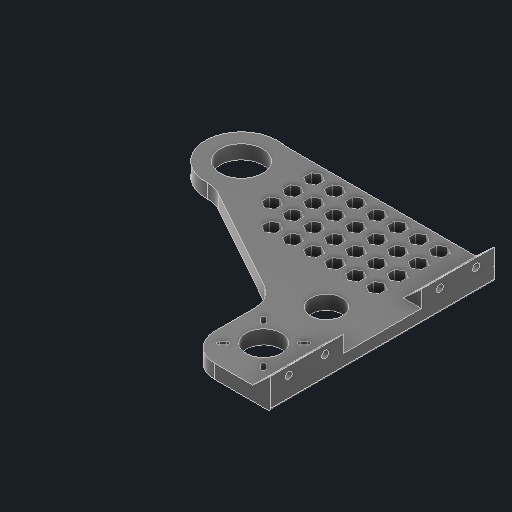
# Autodesk Inventor part: Holder
Saved by Autodesk Inventor 2023 (Build 270158000, 158)
## iProperties
Created: 2023-11-13
Part Number: Holder
Material: Acetal Resin, Black
Document SubType Name: Modeling
Designer: danie
Density: 1.425 g/cm^3
Appearance: Smooth - Black
Author: danie
Autodesk Inventor part; units mm, degrees
ref_plane "YZ Plane" through (0, 0, 0) normal (1, 0, 0) x (0, 1, 0)
ref_plane "XZ Plane" through (0, 0, 0) normal (0, 1, 0) x (-1, 0, 0)
ref_plane "XY Plane" through (0, 0, 0) normal (0, 0, 1) x (1, 0, 0)
sketch "Sketch1" plane through (0, 0, 0) normal (0, 1, 0) x (-1, 0, 0)
  circle A0 centre (35, -30) radius 12.6754
  line L0 (47.071, -15.7062) -> (49.606, -13.1712)
  arc A1 (47.071, -15.7062) -> (49.301, -17.9217) centre (48.1824, -16.8176) ccw
  line L1 (51.8288, -15.394) -> (49.301, -17.9217)
  arc A2 (51.8288, -15.394) -> (49.606, -13.1712) centre (50.7174, -14.2826) ccw
  arc A3 (20.394, -13.1712) -> (18.2539, -15.471) centre (19.2826, -14.2826) ccw
  line L2 (20.394, -13.1712) -> (22.929, -15.7062)
  line L3 (20.6292, -17.8463) -> (18.2539, -15.471)
  arc A4 (20.6292, -17.8463) -> (22.929, -15.7062) centre (21.8176, -16.8176) ccw
  arc A5 (22.929, -44.2938) -> (20.7062, -42.071) centre (21.8176, -43.1824) ccw
  line L4 (22.929, -44.2938) -> (20.394, -46.8288)
  line L5 (18.1712, -44.606) -> (20.7062, -42.071)
  arc A6 (18.1712, -44.606) -> (20.394, -46.8288) centre (19.2826, -45.7174) ccw
  arc A7 (49.606, -46.8288) -> (51.8288, -44.606) centre (50.7174, -45.7174) ccw
  line L6 (49.2938, -42.071) -> (51.8288, -44.606)
  line L7 (49.606, -46.8288) -> (47.071, -44.2938)
  arc A8 (49.2938, -42.071) -> (47.071, -44.2938) centre (48.1824, -43.1824) ccw
  line L8 (0, 0) -> (60, 0)
  line L9 (60, 0) -> (60, -120)
  line L10 (60, -120) -> (0, -120)
  line L11 (0, -120) -> (0, 0)
  line L12 (60, -60) -> (0, -60)
  line L13 (60, -60) -> (150, -110)
  line L14 (150, -110) -> (150, -160)
  line L15 (150, -160) -> (0, -160)
  line L16 (0, -160) -> (0, -120)
  arc A9 (150, -160) -> (150, -110) centre (155.9349, -135) ccw
  circle A10 centre (155.9349, -135) radius 15.25
  line L17 (35, -30) -> (35, -120)
  circle A11 centre (35, -75) radius 11.25
  point P0 (35, -30)
  point P1 (150, -135)
  point P2 (0, -140)
  point P3 (30, -60)
  dimension "d0" = 60
  dimension "d1" = 120
  dimension "d2" = 13.1824
  dimension "d3" = 15.7174
  dimension "d4" = 13.1824
  dimension "d5" = 15.7174
  dimension "d6" = 13.1824
  dimension "d7" = 15.7174
  dimension "d8" = 13.1824
  dimension "d9" = 15.7174
  dimension "d10" = 13.1824
  dimension "d11" = 15.7174
  dimension "d12" = 13.1824
  dimension "d13" = 15.7174
  dimension "d14" = 13.1824
  dimension "d15" = 15.7174
  dimension "d16" = 13.1824
  dimension "d17" = 15.7174
  dimension "d18" = 30
  dimension "d19" = 25
  dimension "d20" = 50
  dimension "d21" = 150
  dimension "d22" = 30.5
  dimension "d90" = 50
  dimension "d91" = 15
  dimension "d92" = 22.5
  dimension "d101" = 120.9349
  dimension "d102" = 35
  dimension "d103" = 135.001
  dimension "d104" = 60
  dimension "d105" = 155.9349
  constraints: 36 end point, 18 point on circle, 12 centre point, 7 midpoint, 4 perpendicular, 2 parallel, 1 coincident, 1 horizontal, 1 point on line, 1 vertical
  measures "d0" distance between parallel lines of L11 L9
  measures "d1" distance between parallel lines of L10 L8
  measures "d2" horizontal distance of A1.centre point (35, -30)
  measures "d3" horizontal distance of A2.centre point (35, -30)
  measures "d4" horizontal distance of A8.centre point (35, -30)
  measures "d5" horizontal distance of A7.centre point (35, -30)
  measures "d6" horizontal distance of A5.centre point (35, -30)
  measures "d7" horizontal distance of A6.centre point (35, -30)
  measures "d8" horizontal distance of A4.centre point (35, -30)
  measures "d9" horizontal distance of A3.centre point (35, -30)
  measures "d10" horizontal distance of A1.centre point (35, -30)
  measures "d11" horizontal distance of A2.centre point (35, -30)
  measures "d12" horizontal distance of A8.centre L17.start
  measures "d13" horizontal distance of point (35, -30) A7.centre
  measures "d14" horizontal distance of A5.centre point (35, -30)
  measures "d15" horizontal distance of A6.centre point (35, -30)
  measures "d16" horizontal distance of A4.centre point (35, -30)
  measures "d17" horizontal distance of A3.centre point (35, -30)
  measures "d18" distance from line of L12 point (35, -30)
  measures "d19" distance from line of point (35, -30) L9
  measures "d20" distance of L13.end L14.end
  measures "d21" distance from line of L16 point (150, -135)
  measures "d22" diameter of A10
  measures "d90" vertical distance of L12.start L13.end
  measures "d91" vertical distance of point (30, -60) A11.centre
  measures "d92" diameter of A11
  measures "d101" horizontal distance of point (35, -75) A9.centre
  measures "d102" distance from line of L11 point (35, -75)
  measures "d103" distance of A11.centre A9.centre
  measures "d104" vertical distance of A11.centre A10.centre
  measures "d105" distance from line of L16 A10.centre
extrude "Extrusion1" add sketch "Sketch1" along normal blind 10 contours L12 L11 L8 L9 | L12 L9 L10 L17 A11 | L17 A11 L10 L11 L12 | L13 L14 A10 L15 L16 L10 L9 | A9 L14 A10
fillet "Fillet1" radius 20 4 edges at (-60, 5, -60) (-60, 5, 0) (-150, 5, -110) (-150, 5, -160)
sketch "Sketch2" plane through (0, 0, 0) normal (0, 0, 1) x (1, 0, 0)
  line L0 (-40, 0) -> (-40, 10) projected
  line L1 (-40, 0) -> (0, 0) projected
  line L2 (0, 0) -> (0, 10) projected
  line L3 (-40, 10) -> (0, 10) projected
  line L4 (0, 10) -> (0, 22)
  line L5 (-20.6292, 0) -> (-18.2539, 0) projected
  line L6 (-18.2539, 0) -> (-18.2539, 10) projected
  line L7 (-20.6292, 10) -> (-18.2539, 10) projected
  line L8 (-20.6292, 0) -> (-20.6292, 10) projected
  line L9 (0, 22) -> (-13, 10)
  line L10 (0, 10) -> (-147.9967, 10) projected
  dimension "d26" = 12
  dimension "d28" = 13
  constraints: 4 end point, 1 point on line, 1 vertical
  measures "d26" distance of L2.end L4.end
  measures "d28" horizontal distance of L4.end L9.end
extrude "Extrusion2" add sketch "Sketch2" against normal blind 160.25 contours L9 L4 L3
sketch "Sketch3" plane through (0, 10, 0) normal (0, 1, 0) x (1, 0, 0)
  line L0 (0, 0) -> (-13, 0) projected
  line L1 (0, 0) -> (0, 160.25) projected
  line L2 (-13, 160.25) -> (0, 160.25) projected
  line L3 (-13, 0) -> (-13, 160) projected
  line L4 (-13, 80) -> (0, 80.125)
  line L5 (-13, 80) -> (-13, 52)
  line L6 (-13, 52) -> (0, 52)
  line L7 (0, 80.125) -> (0, 52)
  line L8 (0, 0) -> (0, 160.25) projected
  line L9 (-13, 80) -> (-13, 108)
  line L10 (-13, 108) -> (0, 108)
  line L11 (0, 108) -> (0, 80.125)
  line L12 (-13, 160) -> (-13, 160.25) projected
  dimension "d31" = 28
  dimension "d32" = 28
  constraints: 14 end point, 4 point on line, 2 collinear, 2 midpoint, 2 perpendicular
  measures "d31" distance of L4.start L5.end
  measures "d32" distance of L4.start L9.end
extrude "Extrusion3" cut sketch "Sketch3" along normal blind 170 contours L6 L3 L4 L1 | L4 L3 L10 L1
sketch "Sketch4" plane through (0, 0, 0) normal (1, 0, 0) x (0, 0, -1)
  line L0 (52, 22) -> (52, 10) projected
  line L1 (52, 16) -> (0, 16)
  line L2 (0, 0) -> (0, 22) projected
  line L3 (108, 10) -> (108, 22) projected
  line L4 (160.25, 10) -> (160.25, 22) projected
  line L5 (0, 22) -> (52, 22) projected
  line L6 (26, 22) -> (26, 16)
  line L7 (108, 22) -> (160.25, 22) projected
  line L8 (26, 16) -> (0, 16)
  line L9 (26, 16) -> (52, 16)
  circle A0 centre (13, 16) radius 2.5
  circle A1 centre (39, 16) radius 2.5
  circle A2 centre (121.1563, 16) radius 2.5
  circle A3 centre (147.2188, 16) radius 2.5
  line L10 (108, 22) -> (108, 10) projected
  line L11 (108, 16) -> (160.25, 16)
  line L12 (134.125, 22) -> (134.125, 16)
  point P0 (170, 12)
  dimension "d35" = 5
  dimension "d36" = 5
  dimension "d37" = 5
  dimension "d84" = 6
  dimension "d85" = 6
  constraints: 12 end point, 9 midpoint, 4 centre point, 3 point on line, 2 collinear, 1 horizontal, 2 other
  measures "d35" diameter of A0
  measures "d36" diameter of A1
  measures "d37" diameter of A2
  measures "d84" distance of point (26, 22) L6.end
  measures "d85" distance between parallel lines of L5 L1
extrude "Extrusion4" cut sketch "Sketch4" against normal blind 170 contours A1 L1 | L1 A1 | A0 L1 | L1 A0 | L11 A2 | A2 L11 | L11 A3 | A3 L11
chamfer "Chamfer1" distance 2 angle 45 4 edges at (-6.5, 16, -10.5) (-6.5, 16, -36.5) (-6.5, 16, -118.6563) (-6.5, 16, -144.7188)
sketch "Sketch5" plane through (0, 10, 0) normal (0, 1, 0) x (1, 0, 0)
  arc A0 (-151.4711, 160.3041) -> (-154.8498, 109.3281) centre (-155.9349, 135) ccw projected
  line L0 (0, 160) -> (-147.9967, 160) projected
  line L1 (-147.9967, 160) -> (0, 160)
  line L2 (-73.9983, 160) -> (-73.9983, 67.7769)
  line L3 (-144.2924, 106.8291) -> (-70.2871, 65.7151) projected
  circle A1 centre (-155.9349, 135) radius 15.25 projected
  line L4 (-140.6849, 135) -> (-73.9983, 135)
  line L5 (-73.9983, 135) -> (0, 135)
  line L6 (0, 0) -> (0, 160) projected
  line L7 (-73.9983, 140.4872) -> (-69.2463, 137.7436)
  line L8 (-69.2463, 137.7436) -> (-69.2463, 132.2564)
  line L9 (-69.2463, 132.2564) -> (-73.9983, 129.5128)
  line L10 (-73.9983, 129.5128) -> (-78.7504, 132.2564)
  line L11 (-78.7504, 132.2564) -> (-78.7504, 137.7436)
  line L12 (-78.7504, 137.7436) -> (-73.9983, 140.4872)
  line L13 (-73.9983, 125.4872) -> (-69.2463, 122.7436)
  line L14 (-69.2463, 122.7436) -> (-69.2463, 117.2564)
  line L15 (-69.2463, 117.2564) -> (-73.9983, 114.5128)
  line L16 (-73.9983, 114.5128) -> (-78.7504, 117.2564)
  line L17 (-78.7504, 122.7436) -> (-73.9983, 125.4872)
  line L18 (-78.7504, 117.2564) -> (-78.7504, 122.7436)
  line L19 (-73.9983, 110.4872) -> (-69.2463, 107.7436)
  line L20 (-69.2463, 107.7436) -> (-69.2463, 102.2564)
  line L21 (-69.2463, 102.2564) -> (-73.9983, 99.5128)
  line L22 (-73.9983, 99.5128) -> (-78.7504, 102.2564)
  line L23 (-78.7504, 107.7436) -> (-73.9983, 110.4872)
  line L24 (-78.7504, 102.2564) -> (-78.7504, 107.7436)
  line L25 (-88.9983, 140.4872) -> (-84.2463, 137.7436)
  line L26 (-84.2463, 137.7436) -> (-84.2463, 132.2564)
  line L27 (-84.2463, 132.2564) -> (-88.9983, 129.5128)
  line L28 (-88.9983, 129.5128) -> (-93.7504, 132.2564)
  line L29 (-93.7504, 137.7436) -> (-88.9983, 140.4872)
  line L30 (-93.7504, 132.2564) -> (-93.7504, 137.7436)
  line L31 (-88.9983, 125.4872) -> (-84.2463, 122.7436)
  line L32 (-84.2463, 122.7436) -> (-84.2463, 117.2564)
  line L33 (-84.2463, 117.2564) -> (-88.9983, 114.5128)
  line L34 (-88.9983, 114.5128) -> (-93.7504, 117.2564)
  line L35 (-93.7504, 122.7436) -> (-88.9983, 125.4872)
  line L36 (-93.7504, 117.2564) -> (-93.7504, 122.7436)
  line L37 (-88.9983, 110.4872) -> (-84.2463, 107.7436)
  line L38 (-84.2463, 107.7436) -> (-84.2463, 102.2564)
  line L39 (-84.2463, 102.2564) -> (-88.9983, 99.5128)
  line L40 (-88.9983, 99.5128) -> (-93.7504, 102.2564)
  line L41 (-93.7504, 107.7436) -> (-88.9983, 110.4872)
  line L42 (-93.7504, 102.2564) -> (-93.7504, 107.7436)
  line L43 (-103.9983, 140.4872) -> (-99.2463, 137.7436)
  line L44 (-99.2463, 137.7436) -> (-99.2463, 132.2564)
  line L45 (-99.2463, 132.2564) -> (-103.9983, 129.5128)
  line L46 (-103.9983, 129.5128) -> (-108.7504, 132.2564)
  line L47 (-108.7504, 137.7436) -> (-103.9983, 140.4872)
  line L48 (-108.7504, 132.2564) -> (-108.7504, 137.7436)
  line L49 (-103.9983, 125.4872) -> (-99.2463, 122.7436)
  line L50 (-99.2463, 122.7436) -> (-99.2463, 117.2564)
  line L51 (-99.2463, 117.2564) -> (-103.9983, 114.5128)
  line L52 (-103.9983, 114.5128) -> (-108.7504, 117.2564)
  line L53 (-108.7504, 122.7436) -> (-103.9983, 125.4872)
  line L54 (-108.7504, 117.2564) -> (-108.7504, 122.7436)
  line L55 (-103.9983, 110.4872) -> (-99.2463, 107.7436)
  line L56 (-99.2463, 107.7436) -> (-99.2463, 102.2564)
  line L57 (-99.2463, 102.2564) -> (-103.9983, 99.5128)
  line L58 (-103.9983, 99.5128) -> (-108.7504, 102.2564)
  line L59 (-108.7504, 107.7436) -> (-103.9983, 110.4872)
  line L60 (-108.7504, 102.2564) -> (-108.7504, 107.7436)
  line L61 (-78.7504, 152.7436) -> (-73.9983, 155.4872)
  line L62 (-78.7504, 147.2564) -> (-78.7504, 152.7436)
  line L63 (-73.9983, 144.5128) -> (-78.7504, 147.2564)
  line L64 (-69.2463, 147.2564) -> (-73.9983, 144.5128)
  line L65 (-69.2463, 152.7436) -> (-69.2463, 147.2564)
  line L66 (-73.9983, 155.4872) -> (-69.2463, 152.7436)
  line L67 (-63.7504, 137.7436) -> (-58.9983, 140.4872)
  line L68 (-63.7504, 132.2564) -> (-63.7504, 137.7436)
  line L69 (-58.9983, 129.5128) -> (-63.7504, 132.2564)
  line L70 (-54.2463, 132.2564) -> (-58.9983, 129.5128)
  line L71 (-54.2463, 137.7436) -> (-54.2463, 132.2564)
  line L72 (-58.9983, 140.4872) -> (-54.2463, 137.7436)
  line L73 (-63.7504, 152.7436) -> (-58.9983, 155.4872)
  line L74 (-63.7504, 147.2564) -> (-63.7504, 152.7436)
  line L75 (-58.9983, 144.5128) -> (-63.7504, 147.2564)
  line L76 (-54.2463, 147.2564) -> (-58.9983, 144.5128)
  line L77 (-54.2463, 152.7436) -> (-54.2463, 147.2564)
  line L78 (-58.9983, 155.4872) -> (-54.2463, 152.7436)
  line L79 (-48.7504, 137.7436) -> (-43.9983, 140.4872)
  line L80 (-48.7504, 132.2564) -> (-48.7504, 137.7436)
  line L81 (-43.9983, 129.5128) -> (-48.7504, 132.2564)
  line L82 (-39.2463, 132.2564) -> (-43.9983, 129.5128)
  line L83 (-39.2463, 137.7436) -> (-39.2463, 132.2564)
  line L84 (-43.9983, 140.4872) -> (-39.2463, 137.7436)
  line L85 (-48.7504, 152.7436) -> (-43.9983, 155.4872)
  line L86 (-48.7504, 147.2564) -> (-48.7504, 152.7436)
  line L87 (-43.9983, 144.5128) -> (-48.7504, 147.2564)
  line L88 (-39.2463, 147.2564) -> (-43.9983, 144.5128)
  line L89 (-39.2463, 152.7436) -> (-39.2463, 147.2564)
  line L90 (-43.9983, 155.4872) -> (-39.2463, 152.7436)
  line L91 (-33.7504, 137.7436) -> (-28.9983, 140.4872)
  line L92 (-33.7504, 132.2564) -> (-33.7504, 137.7436)
  line L93 (-28.9983, 129.5128) -> (-33.7504, 132.2564)
  line L94 (-24.2463, 132.2564) -> (-28.9983, 129.5128)
  line L95 (-24.2463, 137.7436) -> (-24.2463, 132.2564)
  line L96 (-28.9983, 140.4872) -> (-24.2463, 137.7436)
  line L97 (-33.7504, 152.7436) -> (-28.9983, 155.4872)
  line L98 (-33.7504, 147.2564) -> (-33.7504, 152.7436)
  line L99 (-28.9983, 144.5128) -> (-33.7504, 147.2564)
  line L100 (-24.2463, 147.2564) -> (-28.9983, 144.5128)
  line L101 (-24.2463, 152.7436) -> (-24.2463, 147.2564)
  line L102 (-28.9983, 155.4872) -> (-24.2463, 152.7436)
  line L103 (-93.7504, 147.2564) -> (-93.7504, 152.7436)
  line L104 (-88.9983, 144.5128) -> (-93.7504, 147.2564)
  line L105 (-93.7504, 152.7436) -> (-88.9983, 155.4872)
  line L106 (-88.9983, 155.4872) -> (-84.2463, 152.7436)
  line L107 (-84.2463, 152.7436) -> (-84.2463, 147.2564)
  line L108 (-84.2463, 147.2564) -> (-88.9983, 144.5128)
  line L109 (-108.7504, 147.2564) -> (-108.7504, 152.7436)
  line L110 (-103.9983, 144.5128) -> (-108.7504, 147.2564)
  line L111 (-108.7504, 152.7436) -> (-103.9983, 155.4872)
  line L112 (-103.9983, 155.4872) -> (-99.2463, 152.7436)
  line L113 (-99.2463, 152.7436) -> (-99.2463, 147.2564)
  line L114 (-99.2463, 147.2564) -> (-103.9983, 144.5128)
  line L115 (-63.7504, 122.7436) -> (-58.9983, 125.4872)
  line L116 (-63.7504, 117.2564) -> (-63.7504, 122.7436)
  line L117 (-58.9983, 114.5128) -> (-63.7504, 117.2564)
  line L118 (-54.2463, 117.2564) -> (-58.9983, 114.5128)
  line L119 (-54.2463, 122.7436) -> (-54.2463, 117.2564)
  line L120 (-58.9983, 125.4872) -> (-54.2463, 122.7436)
  line L121 (-48.7504, 122.7436) -> (-43.9983, 125.4872)
  line L122 (-48.7504, 117.2564) -> (-48.7504, 122.7436)
  line L123 (-43.9983, 114.5128) -> (-48.7504, 117.2564)
  line L124 (-39.2463, 117.2564) -> (-43.9983, 114.5128)
  line L125 (-39.2463, 122.7436) -> (-39.2463, 117.2564)
  line L126 (-43.9983, 125.4872) -> (-39.2463, 122.7436)
  line L127 (-33.7504, 122.7436) -> (-28.9983, 125.4872)
  line L128 (-33.7504, 117.2564) -> (-33.7504, 122.7436)
  line L129 (-28.9983, 114.5128) -> (-33.7504, 117.2564)
  line L130 (-24.2463, 117.2564) -> (-28.9983, 114.5128)
  line L131 (-24.2463, 122.7436) -> (-24.2463, 117.2564)
  line L132 (-28.9983, 125.4872) -> (-24.2463, 122.7436)
  line L133 (-63.7504, 107.7436) -> (-58.9983, 110.4872)
  line L134 (-63.7504, 102.2564) -> (-63.7504, 107.7436)
  line L135 (-58.9983, 99.5128) -> (-63.7504, 102.2564)
  line L136 (-54.2463, 102.2564) -> (-58.9983, 99.5128)
  line L137 (-54.2463, 107.7436) -> (-54.2463, 102.2564)
  line L138 (-58.9983, 110.4872) -> (-54.2463, 107.7436)
  line L139 (-48.7504, 107.7436) -> (-43.9983, 110.4872)
  line L140 (-48.7504, 102.2564) -> (-48.7504, 107.7436)
  line L141 (-43.9983, 99.5128) -> (-48.7504, 102.2564)
  line L142 (-39.2463, 102.2564) -> (-43.9983, 99.5128)
  line L143 (-39.2463, 107.7436) -> (-39.2463, 102.2564)
  line L144 (-43.9983, 110.4872) -> (-39.2463, 107.7436)
  line L145 (-33.7504, 107.7436) -> (-28.9983, 110.4872)
  line L146 (-33.7504, 102.2564) -> (-33.7504, 107.7436)
  line L147 (-28.9983, 99.5128) -> (-33.7504, 102.2564)
  line L148 (-24.2463, 102.2564) -> (-28.9983, 99.5128)
  line L149 (-24.2463, 107.7436) -> (-24.2463, 102.2564)
  line L150 (-28.9983, 110.4872) -> (-24.2463, 107.7436)
  line L151 (-123.7504, 132.2564) -> (-123.7504, 137.7436)
  line L152 (-118.9983, 129.5128) -> (-123.7504, 132.2564)
  line L153 (-114.2463, 137.7436) -> (-114.2463, 132.2564)
  line L154 (-114.2463, 132.2564) -> (-118.9983, 129.5128)
  line L155 (-123.7504, 137.7436) -> (-118.9983, 140.4872)
  line L156 (-118.9983, 140.4872) -> (-114.2463, 137.7436)
  line L157 (-123.7504, 117.2564) -> (-123.7504, 122.7436)
  line L158 (-123.7504, 122.7436) -> (-118.9983, 125.4872)
  line L159 (-114.2463, 122.7436) -> (-114.2463, 117.2564)
  line L160 (-118.9983, 125.4872) -> (-114.2463, 122.7436)
  line L161 (-118.9983, 114.5128) -> (-123.7504, 117.2564)
  line L162 (-114.2463, 117.2564) -> (-118.9983, 114.5128)
  line L163 (-114.2463, 147.2564) -> (-118.9983, 144.5128)
  line L164 (-114.2463, 152.7436) -> (-114.2463, 147.2564)
  line L165 (-118.9983, 144.5128) -> (-123.7504, 147.2564)
  line L166 (-118.9983, 155.4872) -> (-114.2463, 152.7436)
  line L167 (-123.7504, 147.2564) -> (-123.7504, 152.7436)
  line L168 (-123.7504, 152.7436) -> (-118.9983, 155.4872)
  point P0 (-73.9983, 120)
  point P1 (-73.9983, 120)
  point P2 (-73.9983, 105)
  point P3 (-73.9983, 105)
  point P4 (-88.9983, 135)
  point P5 (-88.9983, 135)
  point P6 (-88.9983, 120)
  point P7 (-88.9983, 120)
  point P8 (-88.9983, 105)
  point P9 (-88.9983, 105)
  point P10 (-103.9983, 135)
  point P11 (-103.9983, 135)
  point P12 (-103.9983, 120)
  point P13 (-103.9983, 120)
  point P14 (-103.9983, 105)
  point P15 (-103.9983, 105)
  point P16 (-108.7504, 105)
  point P17 (-118.9983, 135)
  point P18 (-118.9983, 135)
  point P19 (-118.9983, 120)
  point P20 (-118.9983, 120)
  dimension "d88" = 30.5
  dimension "d46" = 15
  dimension "d49" = 15
  dimension "d54" = 15
  dimension "d57" = 15
  dimension "d62" = 15
  dimension "d69" = 15
  dimension "d76" = 15
  dimension "d83" = 155.9349
  dimension "d89" = 9.5041
  dimension "d93" = 25
  dimension "d96" = 15
  constraints: 332 end point, 11 coincident, 6 horizontal, 5 point on line, 3 midpoint, 3 vertical, 2 collinear, 1 horizontal alignment, 1 perpendicular, 345 other
  measures "d46" distance of point (-73.998, 135) point (-73.998, 120)
  measures "d49" distance of point (-73.998, 135) point (-88.998, 135)
  measures "d54" distance of L11.end L61.start
  measures "d57" distance of L11.end L67.start
  measures "d62" distance of L62.start L103.start
  measures "d69" distance of L17.start L115.start
  measures "d76" distance of L23.start L133.start
  measures "d83" distance from line of L6 A0.centre
  measures "d89" distance from line of L56 point (-108.75, 105)
  measures "d93" distance of point (-73.998, 160) L4.end
  measures "d96" distance of point (-103.998, 135) point (-118.998, 135)
extrude "Extrusion5" cut sketch "Sketch5" against normal blind 15 contours L19 L20 L21 L2 | L2 L22 L24 L23 | L13 L14 L15 L2 | L2 L16 L18 L17 | L153 L154 L152 L151 L4 | L4 L151 L155 L156 L153 | L44 L45 L46 L48 L4 | L4 L48 L47 L43 L44 | L26 L27 L28 L30 L4 | L4 L30 L29 L25 L26 | L66 L65 L64 L2 | L2 L63 L62 L61 | L95 L94 L93 L92 L5 | L5 L92 L91 L96 L95 | L7 L8 L5 L2 | L2 L4 L11 L12 | L83 L82 L81 L80 L5 | L5 L80 L79 L84 L83 | L5 L8 L9 L2 | L2 L10 L11 L4 | L71 L70 L69 L68 L5 | L5 L68 L67 L72 L71 | L31 L32 L33 L34 L36 L35 | L37 L38 L39 L40 L42 L41 | L49 L50 L51 L52 L54 L53 | L55 L56 L57 L58 L60 L59 | L73 L78 L77 L76 L75 L74 | L85 L90 L89 L88 L87 L86 | L97 L102 L101 L100 L99 L98 | L103 L105 L106 L107 L108 L104 | L109 L111 L112 L113 L114 L110 | L115 L120 L119 L118 L117 L116 | L121 L126 L125 L124 L123 L122 | L127 L132 L131 L130 L129 L128 | L133 L138 L137 L136 L135 L134 | L139 L144 L143 L142 L141 L140 | L145 L150 L149 L148 L147 L146 | L157 L158 L160 L159 L162 L161 | L163 L165 L167 L168 L166 L164
fillet "Fillet2" radius 2 1 edges at (0, 0, -80)
body "Solid1"
